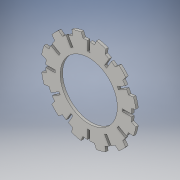
# Autodesk Inventor part: gears big
Saved by Autodesk Inventor 2016 (Build 200138000, 138)
## iProperties
Created: 2017-02-08
Part Number: gears big
Material: Generic
Document SubType Name: Modeling
Designer: jwillauer
Density: 1 g/cm^3
Appearance: Default
Author: jwillauer
Autodesk Inventor part; units mm, degrees
ref_plane "YZ Plane" through (0, 0, 0) normal (1, 0, 0) x (0, 1, 0)
ref_plane "XZ Plane" through (0, 0, 0) normal (0, 1, 0) x (-1, 0, 0)
ref_plane "XY Plane" through (0, 0, 0) normal (0, 0, 1) x (1, 0, 0)
sketch "Sketch1" plane through (0, 0, 0) normal (0, 0, 1) x (1, 0, 0)
  circle A0 centre (0, 0) radius 38.1
  line L0 (1.651, 44.8105) -> (-1.651, 44.8105)
  line L1 (7.7694, 56.6194) -> (10.3029, 62.6586)
  line L2 (-7.5833, 56.6446) -> (-10.0588, 62.6983)
  line L3 (1.651, 57.1261) -> (1.651, 44.8105)
  line L4 (-1.651, 44.8105) -> (-1.651, 57.1261)
  arc A1 (-1.651, 57.1261) -> (-7.5833, 56.6446) centre (0, 0) ccw
  arc A2 (7.7694, 56.6194) -> (1.651, 57.1261) centre (0, 0) ccw
  line L5 (0, 0) -> (0, 48.7919)
  line L6 (-20.9755, 39.6326) -> (-23.8351, 37.9816)
  line L7 (-21.5813, 52.9185) -> (-22.4067, 59.4154)
  line L8 (-34.8897, 45.264) -> (-40.0603, 49.2689)
  line L9 (-27.1333, 50.2982) -> (-20.9755, 39.6326)
  line L10 (-23.8351, 37.9816) -> (-29.9929, 48.6472)
  arc A3 (-29.9929, 48.6472) -> (-34.8897, 45.264) centre (0, 0) ccw
  arc A4 (-21.5813, 52.9185) -> (-27.1333, 50.2982) centre (0, 0) ccw
  line L11 (0, 0) -> (-24.396, 42.2551)
  line L12 (-37.9816, 23.8351) -> (-39.6326, 20.9755)
  line L13 (-45.1492, 35.0382) -> (-49.1125, 40.2519)
  line L14 (-52.8474, 21.755) -> (-59.3277, 22.638)
  line L15 (-48.6472, 29.9929) -> (-37.9816, 23.8351)
  line L16 (-39.6326, 20.9755) -> (-50.2982, 27.1333)
  arc A5 (-50.2982, 27.1333) -> (-52.8474, 21.755) centre (0, 0) ccw
  arc A6 (-45.1492, 35.0382) -> (-48.6472, 29.9929) centre (0, 0) ccw
  line L17 (0, 0) -> (-42.2551, 24.396)
  line L18 (-44.8105, 1.651) -> (-44.8105, -1.651)
  line L19 (-56.6194, 7.7694) -> (-62.6586, 10.3029)
  line L20 (-56.6446, -7.5833) -> (-62.6983, -10.0588)
  line L21 (-57.1261, 1.651) -> (-44.8105, 1.651)
  line L22 (-44.8105, -1.651) -> (-57.1261, -1.651)
  arc A7 (-57.1261, -1.651) -> (-56.6446, -7.5833) centre (0, 0) ccw
  arc A8 (-56.6194, 7.7694) -> (-57.1261, 1.651) centre (0, 0) ccw
  line L23 (0, 0) -> (-48.7919, 0)
  line L24 (-39.6326, -20.9755) -> (-37.9816, -23.8351)
  line L25 (-52.9185, -21.5813) -> (-59.4154, -22.4067)
  line L26 (-45.264, -34.8897) -> (-49.2689, -40.0603)
  line L27 (-50.2982, -27.1333) -> (-39.6326, -20.9755)
  line L28 (-37.9816, -23.8351) -> (-48.6472, -29.9929)
  arc A9 (-48.6472, -29.9929) -> (-45.264, -34.8897) centre (0, 0) ccw
  arc A10 (-52.9185, -21.5813) -> (-50.2982, -27.1333) centre (0, 0) ccw
  line L29 (0, 0) -> (-42.2551, -24.396)
  line L30 (-23.8351, -37.9816) -> (-20.9755, -39.6326)
  line L31 (-35.0382, -45.1492) -> (-40.2519, -49.1125)
  line L32 (-21.755, -52.8474) -> (-22.638, -59.3277)
  line L33 (-29.9929, -48.6472) -> (-23.8351, -37.9816)
  line L34 (-20.9755, -39.6326) -> (-27.1333, -50.2982)
  arc A11 (-27.1333, -50.2982) -> (-21.755, -52.8474) centre (0, 0) ccw
  arc A12 (-35.0382, -45.1492) -> (-29.9929, -48.6472) centre (0, 0) ccw
  line L35 (0, 0) -> (-24.396, -42.2551)
  line L36 (-1.651, -44.8105) -> (1.651, -44.8105)
  line L37 (-7.7694, -56.6194) -> (-10.3029, -62.6586)
  line L38 (7.5833, -56.6446) -> (10.0588, -62.6983)
  line L39 (-1.651, -57.1261) -> (-1.651, -44.8105)
  line L40 (1.651, -44.8105) -> (1.651, -57.1261)
  arc A13 (1.651, -57.1261) -> (7.5833, -56.6446) centre (0, 0) ccw
  arc A14 (-7.7694, -56.6194) -> (-1.651, -57.1261) centre (0, 0) ccw
  line L41 (0, 0) -> (0, -48.7919)
  line L42 (20.9755, -39.6326) -> (23.8351, -37.9816)
  line L43 (21.5813, -52.9185) -> (22.4067, -59.4154)
  line L44 (34.8897, -45.264) -> (40.0603, -49.2689)
  line L45 (27.1333, -50.2982) -> (20.9755, -39.6326)
  line L46 (23.8351, -37.9816) -> (29.9929, -48.6472)
  arc A15 (29.9929, -48.6472) -> (34.8897, -45.264) centre (0, 0) ccw
  arc A16 (21.5813, -52.9185) -> (27.1333, -50.2982) centre (0, 0) ccw
  line L47 (0, 0) -> (24.396, -42.2551)
  line L48 (37.9816, -23.8351) -> (39.6326, -20.9755)
  line L49 (45.1492, -35.0382) -> (49.1125, -40.2519)
  line L50 (52.8474, -21.755) -> (59.3277, -22.638)
  line L51 (48.6472, -29.9929) -> (37.9816, -23.8351)
  line L52 (39.6326, -20.9755) -> (50.2982, -27.1333)
  arc A17 (50.2982, -27.1333) -> (52.8474, -21.755) centre (0, 0) ccw
  arc A18 (45.1492, -35.0382) -> (48.6472, -29.9929) centre (0, 0) ccw
  line L53 (0, 0) -> (42.2551, -24.396)
  line L54 (44.8105, -1.651) -> (44.8105, 1.651)
  line L55 (56.6194, -7.7694) -> (62.6586, -10.3029)
  line L56 (56.6446, 7.5833) -> (62.6983, 10.0588)
  line L57 (57.1261, -1.651) -> (44.8105, -1.651)
  line L58 (44.8105, 1.651) -> (57.1261, 1.651)
  arc A19 (57.1261, 1.651) -> (56.6446, 7.5833) centre (0, 0) ccw
  arc A20 (56.6194, -7.7694) -> (57.1261, -1.651) centre (0, 0) ccw
  line L59 (0, 0) -> (48.7919, 0)
  line L60 (39.6326, 20.9755) -> (37.9816, 23.8351)
  line L61 (52.9185, 21.5813) -> (59.4154, 22.4067)
  line L62 (45.264, 34.8897) -> (49.2689, 40.0603)
  line L63 (50.2982, 27.1333) -> (39.6326, 20.9755)
  line L64 (37.9816, 23.8351) -> (48.6472, 29.9929)
  arc A21 (48.6472, 29.9929) -> (45.264, 34.8897) centre (0, 0) ccw
  arc A22 (52.9185, 21.5813) -> (50.2982, 27.1333) centre (0, 0) ccw
  line L65 (0, 0) -> (42.2551, 24.396)
  line L66 (23.8351, 37.9816) -> (20.9755, 39.6326)
  line L67 (35.0382, 45.1492) -> (40.2519, 49.1125)
  line L68 (21.755, 52.8474) -> (22.638, 59.3277)
  line L69 (29.9929, 48.6472) -> (23.8351, 37.9816)
  line L70 (20.9755, 39.6326) -> (27.1333, 50.2982)
  arc A23 (27.1333, 50.2982) -> (21.755, 52.8474) centre (0, 0) ccw
  arc A24 (35.0382, 45.1492) -> (29.9929, 48.6472) centre (0, 0) ccw
  line L71 (0, 0) -> (24.396, 42.2551)
  arc A25 (22.638, 59.3277) -> (10.3029, 62.6586) centre (0, 0) ccw
  arc A26 (49.2689, 40.0603) -> (40.2519, 49.1125) centre (0, 0) ccw
  arc A27 (62.6983, 10.0588) -> (59.4154, 22.4067) centre (0, 0) ccw
  arc A28 (59.3277, -22.638) -> (62.6586, -10.3029) centre (0, 0) ccw
  arc A29 (40.0603, -49.2689) -> (49.1125, -40.2519) centre (0, 0) ccw
  arc A30 (10.0588, -62.6983) -> (22.4067, -59.4154) centre (0, 0) ccw
  arc A31 (-22.638, -59.3277) -> (-10.3029, -62.6586) centre (0, 0) ccw
  arc A32 (-49.2689, -40.0603) -> (-40.2519, -49.1125) centre (0, 0) ccw
  arc A33 (-62.6983, -10.0588) -> (-59.4154, -22.4067) centre (0, 0) ccw
  arc A34 (-59.3277, 22.638) -> (-62.6586, 10.3029) centre (0, 0) ccw
  arc A35 (-10.0588, 62.6983) -> (-22.4067, 59.4154) centre (0, 0) ccw
  arc A36 (-40.0603, 49.2689) -> (-49.1125, 40.2519) centre (0, 0) ccw
  dimension "d2" = 76.2
  dimension "d4" = 45
  dimension "d5" = 3.302
  dimension "d8" = 1.651
  dimension "d11" = 360
  constraints: 144 end point, 72 point on circle, 37 centre point, 16 coincident, 1 parallel, 1 vertical, 227 other
  measures "d2" diameter of A0
  measures "d4" angle of L2 L1
  measures "d5" distance of L0.start L0.end
  measures "d8" distance between parallel lines of L4 L5
extrude "Extrusion2" add sketch "Sketch1" along normal blind 3.302 contours L59 L54 L57 A20 L55 A28 L50 A17 L52 L48 L53 A0 | A0 L65 L60 L63 A22 L61 A27 L56 A19 L58 L54 L59 | A0 L71 L66 L69 A24 L67 A26 L62 A21 L64 L60 L65 | L53 L48 L51 A18 L49 A29 L44 A15 L46 L42 L47 A0 | A0 L5 L0 L3 A2 L1 A25 L68 A23 L70 L66 L71 | L47 L42 L45 A16 L43 A30 L38 A13 L40 L36 L41 A0 | A0 L11 L6 L9 A4 L7 A35 L2 A1 L4 L0 L5 | A0 L17 L12 L15 A6 L13 A36 L8 A3 L10 L6 L11 | A0 L23 L18 L21 A8 L19 A34 L14 A5 L16 L12 L17 | A0 L29 L24 L27 A10 L25 A33 L20 A7 L22 L18 L23 | A0 L35 L30 L33 A12 L31 A32 L26 A9 L28 L24 L29 | A0 L41 L36 L39 A14 L37 A31 L32 A11 L34 L30 L35
equation "\"d8\" = 0.5 * d5"
equation "\"d13\" = d5"
body "Solid2"
